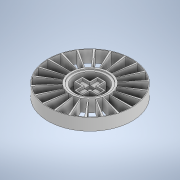
# Autodesk Inventor part: Capsule_Design_Final
Saved by Autodesk Inventor 2022 (Build 260153000, 153)
## iProperties
Created: 2023-02-21
Part Number: Capsule_Design_Final
Material: Generic
Document SubType Name: Modeling
Designer: zarek
Density: 1 g/cm^3
Appearance: Default
Author: zarek
Autodesk Inventor part; units mm, degrees
ref_plane "YZ Plane" through (0, 0, 0) normal (1, 0, 0) x (0, 1, 0)
sketch "Sketch1" plane through (0, 0, 0) normal (0, 1, 0) x (-1, 0, 0)
  circle A0 centre (0, 0) radius 88.9
  dimension "d0" = 177.8
  constraints: 1 centre point, 1 coincident
  measures "d0" diameter of A0
extrude "Extrusion1" add sketch "Sketch1" along normal blind 25.4
sketch "Sketch2" plane through (0, 25.4, 0) normal (0, 1, 0) x (1, 0, 0)
  circle A0 centre (0, 0) radius 87.4
  line L0 (0, 0) -> (-10.8342, 88.2374)
  circle A1 centre (0, 0) radius 88.9 projected
  line L1 (0, 0) -> (10.8342, 88.2374)
  circle A2 centre (0, 0) radius 34.925
  line L2 (0, 0) -> (0, 88.9)
  circle A3 centre (0, 0) radius 41.275
  point P0 (-4.2563, 34.6647)
  point P1 (4.2563, 34.6647)
  point P2 (10.6514, 86.7485)
  point P3 (-10.6514, 86.7485)
  point P4 (-5.0302, 40.9673)
  point P5 (5.0302, 40.9673)
  dimension "d3" = 174.8
  dimension "d4" = 69.85
  dimension "d10" = 14
  dimension "d11" = 7
  dimension "d45" = 82.55
  constraints: 6 end point, 3 centre point, 3 coincident, 3 point on circle, 1 vertical
  measures "d3" diameter of A0
  measures "d4" diameter of A2
  measures "d10" angle of L1 L0
  measures "d11" angle of L1 L2
  measures "d45" diameter of A3
extrude "Extrusion2" cut sketch "Sketch2" against normal blind 25.4 contours L1 A3 L2 A0 | A0 L2 A3 L0
pattern_circular "Circular Pattern1" count 22 over 360 about axis through (0, 0, 0) along (0, 1, 0) of "Extrusion2"
sketch "Sketch4" plane through (0, 25.4, 0) normal (0, 1, 0) x (1, 0, 0)
  circle A0 centre (0, 0) radius 32.425
  dimension "d16" = 64.85
  constraints: 1 centre point, 1 coincident
  measures "d16" diameter of A0
extrude "Extrusion3" cut sketch "Sketch4" against normal blind 20.4
ref_plane "Work Plane1" through (0, 5, 0) normal (0, 1, 0) x (1, 0, 0)
sketch "Sketch5" plane through (0, 5, 0) normal (0, 1, 0) x (1, 0, 0)
  line L0 (0, 0) -> (0, 25)
  line L1 (0, 0) -> (-25, 0)
  line L2 (0, 0) -> (0, -25)
  line L3 (0, 0) -> (25, 0)
  line L4 (25, 0) -> (25, -9)
  line L5 (0, -25) -> (9, -25)
  line L6 (9, -25) -> (9, -9)
  line L7 (9, -9) -> (25, -9)
  line L8 (0, -25) -> (-9, -25)
  line L9 (-9, -25) -> (-9, -9)
  line L10 (-9, -9) -> (-25, -9)
  line L11 (-25, -9) -> (-25, 0)
  line L12 (-25, 0) -> (-25, 9)
  line L13 (-25, 9) -> (-9, 9)
  line L14 (-9, 9) -> (-9, 25)
  line L15 (-9, 25) -> (0, 25)
  line L16 (9, 25) -> (0, 25)
  line L17 (9, 25) -> (9, 9)
  line L18 (9, 9) -> (25, 9)
  line L19 (25, 9) -> (25, 0)
  dimension "d65" = 25
  dimension "d66" = 25
  dimension "d67" = 25
  dimension "d68" = 25
  dimension "d69" = 9
  dimension "d70" = 9
  dimension "d71" = 9
  dimension "d72" = 9
  dimension "d85" = 9
  dimension "d86" = 9
  dimension "d87" = 9
  dimension "d88" = 9
  constraints: 40 end point, 11 point on line, 8 perpendicular, 3 horizontal, 2 vertical, 1 collinear
  measures "d65" distance of L0.start L0.end
  measures "d66" distance of L0.start L1.end
  measures "d67" distance of L0.start L2.end
  measures "d68" distance of L0.start L3.end
  measures "d69" distance of L3.end L4.end
  measures "d70" distance of L2.end L5.end
  measures "d71" distance of L2.end L8.end
  measures "d72" distance of L1.end L12.end
  measures "d85" distance between parallel lines of L3 L18
  measures "d86" distance between parallel lines of L0 L17
  measures "d87" distance between parallel lines of L14 L0
  measures "d88" distance between parallel lines of L10 L1
extrude "Extrusion4" add sketch "Sketch5" along normal blind 15
ref_plane "Work Plane3" through (0, 15.4, 0) normal (0, 1, 0) x (1, 0, 0)
sketch "Sketch21" plane through (0, 25.4, 0) normal (0, 1, 0) x (1, 0, 0)
  circle A0 centre (0, 0) radius 32.425
  circle A1 centre (0, 0) radius 37.425
  dimension "d51" = 64.85
  dimension "d52" = 74.85
  constraints: 2 centre point, 2 coincident
  measures "d51" diameter of A0
  measures "d52" diameter of A1
extrude "Extrusion8" cut sketch "Sketch21" against normal blind 2
sketch "Sketch23" plane through (0, 0, 0) normal (0, -1, 0) x (1, 0, 0)
  circle A0 centre (0, 0) radius 11
  dimension "d60" = 22
  constraints: 1 centre point, 1 coincident
  measures "d60" diameter of A0
extrude "Extrusion10" cut sketch "Sketch23" against normal blind 7
sketch "Sketch7" plane through (0, 15.4, 0) normal (0, 1, 0) x (1, 0, 0)
  line L0 (-6, 6) -> (6, 6)
  line L1 (6, 6) -> (6, -6)
  line L2 (6, -6) -> (-6, -6)
  line L3 (-6, -6) -> (-6, 6)
  line L4 (-15, 15) -> (15, 15) projected
  line L5 (15, 15) -> (15, -15) projected
  line L6 (-15, -15) -> (-15, 15) projected
  line L7 (15, -15) -> (-15, -15) projected
  point P0 (0, 0)
  dimension "d32" = 9
  dimension "d33" = 9
  dimension "d34" = 9
  dimension "d35" = 9
  constraints: 8 end point, 2 parallel, 1 horizontal, 1 perpendicular
  measures "d32" distance between parallel lines of L0 L4
  measures "d33" distance between parallel lines of L5 L1
  measures "d34" distance between parallel lines of L6 L3
  measures "d35" distance between parallel lines of L7 L2
extrude "Extrusion6" cut sketch "Sketch7" against normal blind 5 contours L0 L1 L2 L3
sketch "Sketch25" plane through (0, 20, 0) normal (0, 1, 0) x (1, 0, 0)
  line L0 (-22, 6) -> (-6, 6)
  line L1 (-6, 6) -> (-6, 22)
  line L2 (-6, 22) -> (6, 22)
  line L3 (6, 22) -> (6, 6)
  line L4 (6, 6) -> (22, 6)
  line L5 (22, 6) -> (22, -6)
  line L6 (22, -6) -> (6, -6)
  line L7 (6, -6) -> (6, -22)
  line L8 (6, -22) -> (-6, -22)
  line L9 (-6, -22) -> (-6, -6)
  line L10 (-22, -6) -> (-6, -6)
  line L11 (-22, -6) -> (-22, 6)
  line L12 (-9, 25) -> (-9, 9) projected
  line L13 (9, 25) -> (-9, 25) projected
  line L14 (9, 9) -> (9, 25) projected
  line L15 (9, 9) -> (25, 9) projected
  line L16 (9, -9) -> (25, -9) projected
  line L17 (25, -9) -> (25, 9) projected
  line L18 (9, -25) -> (9, -9) projected
  line L19 (-9, -25) -> (9, -25) projected
  line L20 (-9, -9) -> (-9, -25) projected
  line L21 (-25, -9) -> (-9, -9) projected
  line L22 (-25, 9) -> (-25, -9) projected
  line L23 (-9, 9) -> (-25, 9) projected
  point P0 (0, 0)
  dimension "d73" = 3
  dimension "d74" = 3
  dimension "d75" = 3
  dimension "d76" = 3
  dimension "d77" = 3
  dimension "d78" = 3
  dimension "d79" = 3
  dimension "d80" = 3
  dimension "d81" = 3
  dimension "d82" = 3
  dimension "d83" = 3
  dimension "d84" = 3
  constraints: 24 end point, 8 perpendicular, 8 point on line, 1 horizontal
  measures "d73" distance between parallel lines of L1 L12
  measures "d74" distance between parallel lines of L2 L13
  measures "d75" distance between parallel lines of L14 L3
  measures "d76" distance between parallel lines of L15 L4
  measures "d77" distance between parallel lines of L16 L6
  measures "d78" distance between parallel lines of L17 L5
  measures "d79" distance between parallel lines of L18 L7
  measures "d80" distance between parallel lines of L19 L8
  measures "d81" distance between parallel lines of L20 L9
  measures "d82" distance between parallel lines of L21 L10
  measures "d83" distance between parallel lines of L22 L11
  measures "d84" distance between parallel lines of L0 L23
extrude "Extrusion11" cut sketch "Sketch25" against normal blind 5 contours L0 L1 L2 L3 L4 L5 L6 L7 L8 L9 L10 L11
equation "\"d11\" = 0.5 * d10"
equation "\"d33\" = d32"
equation "\"d34\" = d32"
equation "\"d35\" = d32"
equation "\"d75\" = d73"
equation "\"d76\" = d73"
equation "\"d77\" = d73"
equation "\"d78\" = d73"
equation "\"d80\" = d73"
equation "\"d83\" = d73"
body "Solid1"
